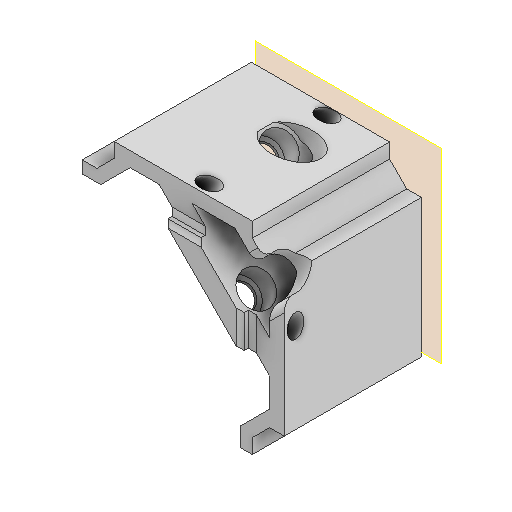
# Autodesk Inventor part: 20_Cube_Insert_Kinematic_Mirror_45_pro_magnetic
Saved by Autodesk Inventor 2022 (Build 260153000, 153)
## iProperties
Created: 2022-01-05
Part Number: 20_Cube_Insert_Kinematic_Mirror_45_pro_magnetic
Material: Generisch
Document SubType Name: Modeling
Designer: diederichbenedict
Density: 1 g/cm^3
Appearance: Vorgabe
Catalog Web Link: isPrinted
Vendor: openUC2
Author: diederichbenedict
Autodesk Inventor part; units mm, degrees
ref_plane "YZ Plane" through (0, 0, 0) normal (1, 0, 0) x (0, 1, 0)
ref_plane "XZ Plane" through (0, 0, 0) normal (0, 1, 0) x (-1, 0, 0)
ref_plane "XY Plane" through (0, 0, 0) normal (0, 0, 1) x (1, 0, 0)
ref_plane "Arbeitsebene1" through (0, 0, 0) normal (0, 0, 1) x (1, 0, 0)
sketch "Skizze1" plane through (0, 0, 0) normal (0, 0, 1) x (1, 0, 0)
  line L0 (14.02, 21.9) -> (-20.02, 21.9)
  line L1 (34.79, 34.79) -> (-34.79, -34.79)
  line L2 (14.02, 21.9) -> (14.02, 14.02)
  line L3 (14.02, 14.02) -> (10.02, 10.02)
  line L4 (-20.02, 21.9) -> (-1.74, 21.9)
  line L5 (-20.02, 18.2674) -> (-24.2698, 14.02)
  line L6 (8.7191, 8.7191) -> (6.14, 6.14)
  line L7 (-20.02, 14.02) -> (-20.02, 18.2) projected
  line L8 (-20.02, 18.2) -> (14.02, 18.2) construction
  line L9 (14.02, 18.2) -> (14.02, 14.02) projected
  line L10 (14.02, 14.02) -> (18.2698, 14.02) projected
  line L11 (18.2698, 14.02) -> (18.2698, -20.02) projected
  line L12 (18.2698, -20.02) -> (14.02, -20.02) projected
  line L13 (14.02, -20.02) -> (14.02, -24.2) projected
  line L14 (14.02, -24.2) -> (-20.02, -24.2) projected
  line L15 (-20.02, -24.2) -> (-20.02, -20.02) projected
  line L16 (-20.02, -20.02) -> (-24.2698, -20.02) projected
  line L17 (-24.2698, -20.02) -> (-24.2698, 14.02) projected
  line L18 (-24.2698, 14.02) -> (-20.02, 14.02) projected
  line L19 (-23.8273, -20.7803) -> (-20.8134, -23.5239) projected
  arc A0 (-20.65, -23.8937) -> (-20.8134, -23.5239) centre (-21.15, -23.8937) ccw projected
  line L20 (-20.65, -23.8937) -> (-20.65, -26.25) projected
  arc A1 (-21.15, -26.75) -> (-20.65, -26.25) centre (-21.15, -26.25) ccw projected
  line L21 (-21.15, -26.75) -> (-26.25, -26.75) projected
  arc A2 (-26.75, -26.25) -> (-26.25, -26.75) centre (-26.25, -26.25) ccw projected
  line L22 (-26.75, -26.25) -> (-26.75, -21.15) projected
  arc A3 (-26.25, -20.65) -> (-26.75, -21.15) centre (-26.25, -21.15) ccw projected
  line L23 (-26.25, -20.65) -> (-24.1639, -20.65) projected
  arc A4 (-23.8273, -20.7803) -> (-24.1639, -20.65) centre (-24.1639, -21.15) ccw projected
  line L24 (20.75, 20.25) -> (20.75, 15.15) projected
  arc A5 (20.25, 14.65) -> (20.75, 15.15) centre (20.25, 15.15) ccw projected
  line L25 (20.25, 14.65) -> (17.8937, 14.65) projected
  arc A6 (17.5239, 14.8134) -> (17.8937, 14.65) centre (17.8937, 15.15) ccw projected
  line L26 (17.5239, 14.8134) -> (14.7803, 17.8273) projected
  arc A7 (14.65, 18.1639) -> (14.7803, 17.8273) centre (15.15, 18.1639) ccw projected
  line L27 (14.65, 18.1639) -> (14.65, 20.25) projected
  arc A8 (15.15, 20.75) -> (14.65, 20.25) centre (15.15, 20.25) ccw projected
  line L28 (15.15, 20.75) -> (20.25, 20.75) projected
  arc A9 (20.75, 20.25) -> (20.25, 20.75) centre (20.25, 20.25) ccw projected
  arc A10 (21.9, 19.9) -> (19.9, 21.9) centre (19.9, 19.9) ccw projected
  line L29 (19.9, 21.9) -> (-20.02, 21.9) projected
  line L30 (-20.02, 21.9) -> (-20.02, 18.2686) projected
  line L31 (-24.2711, 14.02) -> (-20.02, 18.2686) projected
  line L32 (-24.2711, 14.02) -> (-27.9, 14.02) projected
  line L33 (-27.9, 14.02) -> (-27.9, -25.9) projected
  arc A11 (-27.9, -25.9) -> (-25.9, -27.9) centre (-25.9, -25.9) ccw projected
  line L34 (-25.9, -27.9) -> (14.02, -27.9) projected
  line L35 (14.02, -27.9) -> (14.02, -24.2686) projected
  line L36 (18.2711, -20.02) -> (14.02, -24.2686) projected
  line L37 (18.2711, -20.02) -> (21.9, -20.02) projected
  line L38 (21.9, -20.02) -> (21.9, 19.9) projected
  line L39 (-20.02, 18.2686) -> (14.02, 18.2686)
  line L40 (-20.02, 18.2686) -> (14.02, 18.2686) construction
  line L41 (14.02, 18.2686) -> (16.1443, 16.1443)
  line L42 (16.1443, 16.1443) -> (14.02, 14.02)
  line L43 (14.02, 14.02) -> (9.7714, 18.2686)
  line L44 (-16.0848, 18.2) -> (-16.0848, 18.2686)
  line L45 (-16.0848, 18.2686) -> (-20.02, 18.2686)
  line L46 (-20.02, 18.2686) -> (-20.02, 18.2)
  line L47 (-27.9, 14.02) -> (-27.9, 11.0221)
  line L48 (-27.9, 11.0221) -> (-23.3354, 11.0221)
  line L49 (8.7191, 8.7191) -> (-0.8305, 18.2686)
  line L50 (8.7191, 8.7191) -> (22.2242, 8.7191) construction
  line L51 (4.6555, 4.6555) -> (-8.9576, 18.2686)
  line L52 (4.6555, 4.6555) -> (23.9073, 4.6555) construction
  line L53 (-16.0848, 18.2686) -> (-23.3354, 11.0221)
  line L54 (-16.0848, 18.2686) -> (-5.8338, 18.2686) construction
  line L55 (-20.02, 18.2) -> (-20.02, 21.9)
  line L56 (-24.2698, 14.02) -> (-27.9, 14.02)
  point P0 (0, 0)
  point P1 (-8.9576, 18.2686)
  point P2 (4.6555, 4.6555)
  point P3 (-24.2698, 11.0221)
  dimension "d41" = 0
  dimension "d42" = 135
  dimension "d43" = 2.9979
  dimension "d44" = 135
  dimension "d45" = 135
  dimension "d46" = 5.747
  dimension "d47" = 135.016
  constraints: 50 end point, 10 point on line, 6 horizontal, 4 equal length, 4 parallel, 3 perpendicular, 1 collinear, 1 vertical, 10 other
  measures "d41" distance between parallel lines of L39 L40
  measures "d42" angle of L39 L41
  measures "d43" distance of L47.end L47.start
  measures "d44" angle of L50 L49
  measures "d45" angle of L52 L51
  measures "d47" angle of L53 L54
extrude "Extrusion1" add sketch "Skizze1" along normal blind 33.8 contours L2 L39 L30 L0 | L41 L1 L2 | L2 L43 L39 | L46 L7 L53 L18 L5 | L39 L53 L7 L46 | L49 L1 L51 L39 | L18 L53 L48 L17 | L17 L48 L33 L32
mirror "Spiegeln1" about plane through (4.6555, 4.6555, 0) normal (0.7071068, -0.7071068, 0) of "Extrusion1"
sketch "Skizze3" plane through (16.5235, 15.7652, 0) normal (0.7071068, 0.7071068, 0) x (-0.7071068, 0.7071068, 0)
  line L0 (16.5535, -1.95) -> (-15.4465, -1.95) projected
  line L1 (-18.4465, 1.05) -> (-15.4465, -1.95) projected
  line L2 (-18.4465, 1.05) -> (-18.4465, 33.05) projected
  line L3 (-15.4465, 36.05) -> (-18.4465, 33.05) projected
  line L4 (-15.4465, 36.05) -> (16.5535, 36.05) projected
  line L5 (19.5535, 33.05) -> (16.5535, 36.05) projected
  line L6 (19.5535, 33.05) -> (19.5535, 1.05) projected
  line L7 (11.5535, 33.05) -> (19.5535, 33.05) projected
  line L8 (16.5535, 36.05) -> (19.5535, 33.05) projected
  line L9 (-15.4465, 36.05) -> (16.5535, 36.05) projected
  line L10 (-18.4465, 33.05) -> (-15.4465, 36.05) projected
  line L11 (-18.4465, 1.05) -> (-18.4465, 33.05) projected
  line L12 (-15.4465, -1.95) -> (-18.4465, 1.05) projected
  line L13 (16.5535, -1.95) -> (-15.4465, -1.95) projected
  line L14 (19.5535, 1.05) -> (16.5535, -1.95) projected
  line L15 (19.5535, 29.05) -> (19.5535, 1.05) projected
  line L16 (19.5535, 29.05) -> (11.5535, 29.05) projected
  line L17 (11.5535, 29.05) -> (11.5535, 33.05) projected
  circle A0 centre (-13.4465, 31.05) radius 2 projected
  circle A1 centre (-13.4465, 31.05) radius 1.45
  circle A2 centre (15.5535, 31.05) radius 1.4
  line L18 (-18.7156, 0) -> (-18.7156, 33.8) projected
  line L19 (-14.9465, 20.05) -> (-14.9465, 14.05) construction
  line L20 (-16.4465, 20.05) -> (-16.4465, 14.05)
  line L21 (-13.4465, 14.05) -> (-13.4465, 20.05)
  arc A3 (-13.4465, 20.05) -> (-16.4465, 20.05) centre (-14.9465, 20.05) ccw
  arc A4 (-16.4465, 14.05) -> (-13.4465, 14.05) centre (-14.9465, 14.05) ccw
  line L22 (3.5535, 32.63) -> (-2.4465, 32.63) construction
  line L23 (3.5535, 34.13) -> (-2.4465, 34.13)
  line L24 (-2.4465, 31.13) -> (3.5535, 31.13)
  arc A5 (3.5535, 31.13) -> (3.5535, 34.13) centre (3.5535, 32.63) ccw
  arc A6 (-2.4465, 34.13) -> (-2.4465, 31.13) centre (-2.4465, 32.63) ccw
  line L25 (-13.4465, 31.05) -> (15.5535, 31.05) construction
  line L26 (15.5535, 31.05) -> (15.5535, 2.05) construction
  line L27 (15.5535, 2.05) -> (-13.4465, 2.05) construction
  line L28 (-13.4465, 2.05) -> (-13.4465, 31.05) construction
  circle A7 centre (-13.4465, 2.05) radius 2
  circle A8 centre (-4.4465, 31.05) radius 4 projected
  circle A9 centre (14.5535, 12.05) radius 4 projected
  line L29 (16.5535, -1.95) -> (19.5535, 1.05) projected
  circle A10 centre (-4.4465, 31.05) radius 3 projected
  circle A11 centre (14.5535, 12.05) radius 3 projected
  circle A12 centre (15.5535, 2.05) radius 1.4
  circle A13 centre (15.5535, 31.05) radius 2
  circle A14 centre (15.5535, 2.05) radius 2
  point P0 (0.5362, 0)
  point P1 (3.5535, 34.13)
  point P2 (-2.4465, 34.13)
  point P3 (-2.4465, 31.13)
  point P4 (3.5535, 31.13)
  point P5 (-16.4465, 14.05)
  point P6 (-13.4465, 14.05)
  point P7 (-13.4465, 20.05)
  point P8 (-16.4465, 20.05)
  point P9 (-11.3665, -1.95)
  point P10 (-14.9465, 17.05)
  point P11 (0.5535, 32.63)
  dimension "d48" = 2.9
  dimension "d49" = 2.8
  dimension "d58" = 29
  dimension "d59" = 29
  dimension "d60" = 4
  dimension "d84" = 4
  dimension "d85" = 4
  dimension "d86" = 4
  constraints: 24 end point, 10 centre point, 8 point on circle, 8 tangent, 4 coincident, 4 parallel, 2 midpoint, 2 perpendicular, 1 horizontal, 1 point on line, 1 vertical
  measures "d48" diameter of A1
  measures "d49" diameter of A2
  measures "d58" distance of L26.end L27.end
  measures "d59" distance of L25.end L26.end
  measures "d60" diameter of A7
  measures "d84" diameter of A0
  measures "d85" diameter of A13
  measures "d86" diameter of A14
extrude "Extrusion2" cut sketch "Skizze3" against normal blind 33.8 contours A13 | A0 | A1 | A2 | A12 | A14
sketch "Skizze7" plane through (18.2686, 14.02, 0) normal (0.7071068, 0.7071068, 0) x (-0.7071068, 0.7071068, 0)
  circle A0 centre (-10.9784, 31.05) radius 1.45 projected
  circle A1 centre (-10.9784, 2.05) radius 2 projected
  point P0 (3.0042, 0)
  point P1 (18.0216, 31.05)
hole "Bohrung2" at (5.5254, 26.7632, 31.05) at (26.0315, 6.2571, 31.05) direction (-0.7071068, -0.7071068, 0) diameter 4.1 end through all
sketch "Skizze9" plane through (-8.9576, 18.2686, 33.8) normal (-0.7071068, -0.7071068, 0) x (-0.7071068, 0.7071068, 0)
  circle A0 centre (-24.2345, 2.75) radius 4 projected
  circle A1 centre (-5.2345, 21.75) radius 4 projected
  line L0 (-35.2345, -2.25) -> (-38.2345, 0.75) projected
  line L1 (-35.2345, -2.25) -> (-3.2345, -2.25) projected
  line L2 (-0.2345, 0.75) -> (-3.2345, -2.25) projected
  line L3 (-0.2345, 0.75) -> (-0.2345, 32.75) projected
  line L4 (-3.2345, 35.75) -> (-0.2345, 32.75) projected
  line L5 (-3.2345, 35.75) -> (-35.2345, 35.75) projected
  line L6 (-38.2345, 32.75) -> (-35.2345, 35.75) projected
  line L7 (-38.2345, 32.75) -> (-38.2345, 0.75) projected
  circle A2 centre (-5.2345, 21.75) radius 3
  circle A3 centre (-24.2345, 2.75) radius 3
  point P0 (-19.2518, 33.8)
  dimension "d70" = 6
  dimension "d71" = 6
  constraints: 2 centre point, 2 coincident
  measures "d70" diameter of A2
  measures "d71" diameter of A3
extrude "Extrusion7" cut sketch "Skizze9" against normal through all contours A2 | A3
sketch "Skizze10" plane through (0, 0, 33.8) normal (0, 0, 1) x (1, 0, 0)
  line L0 (16.6955, 11.3445) -> (19.371, 14.02) projected
  line L1 (18.2686, 14.02) -> (19.371, 14.02) projected
  line L2 (14.02, 18.2686) -> (18.2686, 14.02) projected
  line L3 (14.02, 18.2686) -> (14.02, 21.9) projected
  line L4 (14.02, 21.9) -> (-20.02, 21.9) projected
  line L5 (-20.02, 21.9) -> (-20.02, 18.2686) projected
  line L6 (-20.02, 18.2686) -> (-24.2711, 14.02) projected
  line L7 (-24.2711, 14.02) -> (-27.9, 14.02) projected
  line L8 (-27.9, 14.02) -> (-27.9, 11.0221) projected
  line L9 (-27.9, 11.0221) -> (-23.3354, 11.0221) projected
  line L10 (-23.3354, 11.0221) -> (-16.0848, 18.2686) projected
  line L11 (-16.0848, 18.2686) -> (-8.9576, 18.2686) projected
  line L12 (-8.9576, 18.2686) -> (7.331, 1.98) projected
  line L13 (7.331, 1.98) -> (11.3945, 6.0436) projected
  line L14 (-0.8305, 18.2686) -> (11.3945, 6.0436) projected
  line L15 (-0.8305, 18.2686) -> (9.7714, 18.2686) projected
  line L16 (9.7714, 18.2686) -> (16.6955, 11.3445) projected
  line L17 (21.9, 13.1579) -> (18.2686, 9.5265) projected
  line L18 (18.2686, -0.8305) -> (18.2686, 9.5265) projected
  line L19 (13.0901, 4.348) -> (18.2686, -0.8305) projected
  line L20 (13.0901, 4.348) -> (9.0266, 0.2844) projected
  line L21 (9.0266, 0.2844) -> (18.2686, -8.9576) projected
  line L22 (18.2686, -16.0848) -> (18.2686, -8.9576) projected
  line L23 (11.0221, -23.3354) -> (18.2686, -16.0848) projected
  line L24 (11.0221, -27.9) -> (11.0221, -23.3354) projected
  line L25 (14.02, -27.9) -> (11.0221, -27.9) projected
  line L26 (14.02, -24.2711) -> (14.02, -27.9) projected
  line L27 (18.2686, -20.02) -> (14.02, -24.2711) projected
  line L28 (21.9, -20.02) -> (18.2686, -20.02) projected
  line L29 (21.9, 13.1579) -> (21.9, -20.02) projected
  line L30 (-20.02, 14.0445) -> (14.02, 14.0445) projected
  line L31 (14.02, 14.0445) -> (14.02, -19.9955) projected
  line L32 (-8.9576, 18.2686) -> (7.331, 1.98) projected
  line L33 (7.331, 1.98) -> (9.0266, 0.2844)
  line L34 (13.0901, 4.348) -> (9.0266, 0.2844) projected
  line L35 (13.0901, 4.348) -> (11.3945, 6.0436)
  point P0 (0, 0)
  point P1 (3.3936, 14.0445)
  point P2 (-4.7335, 14.0445)
  point P3 (14.02, -4.709)
  point P4 (14.02, 3.4181)
  constraints: 4 end point, 1 collinear, 1 perpendicular
extrude "Extrusion8" add sketch "Skizze10" along normal blind 3 contours L31 L21 L20 L19 | L14 L13 L12 L30 | L20 L33 L13 L35
chamfer "Fase2" distance 1 angle 45 4 edges at (14.02, -0.6454, 36.8) (14.02, -0.6454, 33.8) (-0.67, 14.0445, 36.8) (-0.67, 14.0445, 33.8)
sketch "Skizze11" plane through (14.02, 18.2686, 0) normal (0.7071068, 0.7071068, 0) x (-0.7071068, 0.7071068, 0)
  arc A0 (-9.1858, 33.8) -> (-8.5762, 28.1085) centre (-7.9869, 31.05) ccw projected
  circle A1 centre (11.0131, 12.05) radius 3 projected
  circle A2 centre (-7.9869, 31.05) radius 4.1
  circle A3 centre (11.0131, 12.05) radius 4.1
  point P0 (-3.0042, 0)
  dimension "d79" = 8.2
  dimension "d80" = 8.2
  constraints: 2 centre point, 2 coincident
  measures "d79" diameter of A2
  measures "d80" diameter of A3
extrude "Extrusion9" cut sketch "Skizze11" along normal mid plane 31 contours A1 | A2 | A3
fillet "Rundung2" radius 2 2 edges at (20.0843, 8.7372, 33.8) (16.4551, 13.7092, 33.8)
sketch "Skizze12" plane through (18.6063, -1.1682, 2.05) normal (0.7071068, 0.7071068, 0) x (-0.7071068, 0.7071068, 0)
  circle A0 centre (28, 10) radius 4.1 projected
  circle A1 centre (29, 29) radius 2.05 projected
  circle A2 centre (29, 0) radius 2 projected
  line L0 (19.5547, -2.05) -> (43.6246, -2.05) projected
  line L1 (43.6246, -2.05) -> (43.6246, 31.75) projected
  line L2 (19.5547, 31.75) -> (43.6246, 31.75) projected
  line L3 (19.5547, -2.05) -> (19.5547, 31.75) projected
  circle A3 centre (28, 10) radius 5
  point P0 (13.9827, -2.05)
  dimension "d87" = 10
  constraints: 1 centre point, 1 coincident
  measures "d87" diameter of A3
extrude "Extrusion10" cut sketch "Skizze12" along normal blind 33.8 contours A0 | A3
